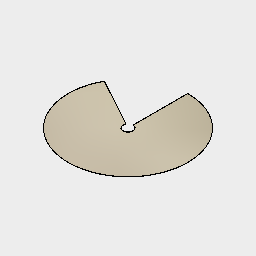
Cone Net Drawing (Autodesk Fusion 360 archive; units mm, degrees)
design "Cone Net"
Autodesk Fusion 360 part; units mm, degrees
sketch "Sketch1" plane through (0, 0, 0) normal (0, 1, 0) x (1, 0, 0)
  circle A0 centre (0, 0) radius 29.886
  line L0 (0, 0) -> (0, 29.886)
  line L1 (0, 0) -> (-26.2076, 14.3643)
  line L2 (0, 0) -> (29.886, 0) construction
  circle A1 centre (0, 0) radius 2.5
  dimension "d10" = 59.772
  dimension "d13" = 61.273
  dimension "d14" = 5
  measures "d10" diameter of A0
  measures "d13" angle of L0 L1
  measures "d14" diameter of A1
extrude "Extrude1" add sketch "Sketch1" along normal blind 0.1 contours A0 L0 L1 A1 picked at (20.6429, -1.5675)
equation "d10 = ( 29.886 * 2 ) * 1 mm"
